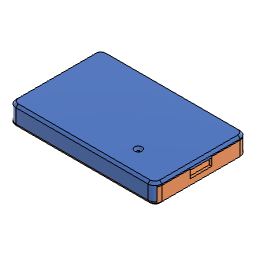
ESP32+Devkit+v4+Case (Autodesk Fusion 360 design; units mm, degrees)
Autodesk Fusion 360 part; units mm, degrees
sketch "Board" plane through (0, 0, 0) normal (0, 0, 1) x (1, 0, 0)
  line L0 (-24.2, 14.1) -> (24.2, 14.1)
  line L1 (24.2, 14.1) -> (24.2, -14.1)
  line L2 (24.2, -14.1) -> (-24.2, -14.1)
  line L3 (-24.2, -14.1) -> (-24.2, 14.1)
  line L4 (-24.2, 14.1) -> (24.2, -14.1) construction
  line L5 (24.2, 14.1) -> (-24.2, -14.1) construction
  line L6 (18.3, 3.8) -> (25, 3.8)
  line L7 (25, 3.8) -> (25, -3.8)
  line L8 (25, -3.8) -> (18.3, -3.8)
  line L9 (18.3, -3.8) -> (18.3, 3.8)
  line L10 (-24.2, 0) -> (24.2, 0) construction
  line L11 (-23.4, 7.9) -> (-5.9, 7.9)
  line L12 (-5.9, 7.9) -> (-5.9, -7.9)
  line L13 (-5.9, -7.9) -> (-23.4, -7.9)
  line L14 (-23.4, -7.9) -> (-23.4, 7.9)
  line L15 (-30.2, 9) -> (-23.4, 9)
  line L16 (-23.4, 9) -> (-23.4, -9)
  line L17 (-23.4, -9) -> (-30.2, -9)
  line L18 (-30.2, -9) -> (-30.2, 9)
  line L19 (-24, 14) -> (24, 14)
  line L20 (24, 14) -> (24, 11.6)
  line L21 (24, 11.6) -> (-24, 11.6)
  line L22 (-24, 11.6) -> (-24, 14)
  line L23 (-24, -11.6) -> (24, -11.6)
  line L24 (24, -11.6) -> (24, -14)
  line L25 (24, -14) -> (-24, -14)
  line L26 (-24, -14) -> (-24, -11.6)
  line L27 (10.2, -7.6) -> (12.2, -7.6)
  line L28 (12.2, -7.6) -> (12.2, -8.6)
  line L29 (12.2, -8.6) -> (10.2, -8.6)
  line L30 (10.2, -8.6) -> (10.2, -7.6)
  point P0 (25, 0)
  point P1 (-23.4, 0)
  dimension "d1" = 48.4
  dimension "d2" = 28.2
  dimension "d3" = 7.6
  dimension "d4" = 6.7
  dimension "d5" = 0.8
  dimension "d6" = 17.5
  dimension "d7" = 15.8
  dimension "d8" = 0.8
  dimension "d9" = 18
  dimension "d10" = 6.8
  dimension "d11" = 2.4
  dimension "d12" = 0.1
  dimension "d13" = 0.2
  dimension "d14" = 48
  dimension "d15" = 2.4
  dimension "d16" = 0.1
  dimension "d17" = 0.2
  dimension "d18" = 48
  dimension "d64" = 2
  dimension "d65" = 1
  dimension "d66" = 12
  dimension "d67" = 5.5
  constraint horizontal L0
  constraint perpendicular L0 L1
  constraint parallel L0 L2
  constraint parallel L1 L3
  constraint coincident L4 origin
  constraint coincident L5 origin
  constraint horizontal L6
  constraint vertical L7
  constraint horizontal L8
  constraint vertical L9
  constraint midpoint L3 L10.start
  constraint midpoint L1 L10.end
  constraint midpoint L7 P0
  constraint horizontal L10.end P0
  constraint horizontal L11
  constraint vertical L12
  constraint horizontal L13
  constraint vertical L14
  constraint midpoint L14 P1
  constraint horizontal L10.start P1
  constraint horizontal L15
  constraint vertical L16
  constraint horizontal L17
  constraint vertical L18
  constraint midpoint L14 L16
  constraint horizontal L19
  constraint vertical L20
  constraint horizontal L21
  constraint vertical L22
  constraint horizontal L23
  constraint vertical L24
  constraint horizontal L25
  constraint vertical L26
  constraint horizontal L27
  constraint vertical L28
  constraint horizontal L29
  constraint vertical L30
  measures "d1" distance of L0.start L0.end
  measures "d2" distance of L0.start L2.end
  measures "d3" distance of L6.end L7.end
  measures "d4" distance of L6.start L6.end
  measures "d5" distance of L1 L7
  measures "d6" distance of L11.start L11.end
  measures "d7" distance of L11.start L13.end
  measures "d8" distance of L3 L14
  measures "d9" distance of L15.start L17.end
  measures "d10" distance of L15.start L15.end
  measures "d11" distance of L19.end L20.end
  measures "d12" distance of L0 L19
  measures "d13" distance of L3 L22
  measures "d14" distance of L20.end L21.end
  measures "d15" distance of L23.end L24.end
  measures "d16" distance of L2 L25
  measures "d17" distance of L3 L26
  measures "d18" distance of L23.start L23.end
  measures "d64" distance of L27.start L27.end
  measures "d65" distance of L27.start L29.end
  measures "d66" distance of L1 L28.end
  measures "d67" distance of L2 L28.end
sketch "Case" plane through (0, 0, 0) normal (0, 0, 1) x (1, 0, 0)
  line L0 (-24.2, 14.1) -> (24.2, 14.1) construction
  line L1 (24.2, 14.1) -> (24.2, -14.1) construction
  line L2 (24.2, -14.1) -> (-24.2, -14.1) construction
  line L3 (-24.2, -14.1) -> (-24.2, 14.1) construction
  line L4 (24.4, -14.3) -> (-24.4, -14.3)
  line L5 (-24.4, -14.3) -> (-24.4, 14.3)
  line L6 (-24.4, 14.3) -> (24.4, 14.3)
  line L7 (24.4, 14.3) -> (24.4, -14.3)
  line L8 (25.3, -15.2) -> (-25.3, -15.2)
  line L9 (-25.3, -15.2) -> (-25.3, 15.2)
  line L10 (-25.3, 15.2) -> (25.3, 15.2)
  line L11 (25.3, 15.2) -> (25.3, -15.2)
  line L12 (26.4, -16.3) -> (-26.4, -16.3) construction
  line L13 (-26.4, -16.3) -> (-26.4, 16.3)
  line L14 (-26.4, 16.3) -> (26.4, 16.3) construction
  line L15 (26.4, 16.3) -> (26.4, -16.3) construction
  line L16 (25.3, 15.2) -> (25.3, 16.3)
  line L17 (25.3, -15.2) -> (25.3, -16.3)
  line L18 (25.3, 16.3) -> (-26.4, 16.3)
  line L19 (25.3, -16.3) -> (-26.4, -16.3)
  line L20 (24, 11.6) -> (-24, 11.6) construction
  line L21 (-24, -11.6) -> (24, -11.6) construction
  line L22 (-24.4, -11.4) -> (24.4, -11.4)
  line L23 (-24.4, 11.4) -> (24.4, 11.4)
  dimension "d26" = 0.2
  dimension "d27" = 0.2
  constraint coincident L14 L16.end
  constraint perpendicular L14 L16
  constraint coincident L12 L17.end
  constraint perpendicular L12 L17
  constraint coincident L5 L22.start
  constraint coincident L7 L22.end
  constraint perpendicular L7 L22
  constraint coincident L5 L23.start
  constraint coincident L7 L23.end
  constraint perpendicular L1 L23
  measures "d26" distance of L21 L22
  measures "d27" distance of L20 L23
extrude "Extrude1" add sketch "Case" against normal blind 1.2 contours L5 L7 L22 L23 | L8 L9 L10 L13 L16 L17 L18 L19 | L8 L9 L10 L11 makes body 1 in component "Base"
extrude "Extrude2" add sketch "Case" along normal blind 1.6 contours L8 L9 L10 L11 bodies 1 in component "Base"
sketch "Sketch3" plane through (0, 0, 1.6) normal (0, 0, 1) x (-1, 0, 0) in component "Base"
  line L0 (24.4, -14.3) -> (-24.4, -14.3)
  line L1 (-24.4, -14.3) -> (-24.4, 14.3)
  line L2 (-24.4, 14.3) -> (24.4, 14.3)
  line L3 (24.4, 14.3) -> (24.4, -14.3)
  line L4 (-25.3, -15.2) -> (25.3, -15.2)
  line L5 (25.3, -15.2) -> (25.3, 15.2)
  line L6 (25.3, 15.2) -> (-25.3, 15.2)
  line L7 (-25.3, 15.2) -> (-25.3, -15.2)
  line L8 (-18.3, -3.8) -> (-25, -3.8)
  line L9 (-25, 3.8) -> (-18.3, 3.8)
  line L10 (-25.3, -15.2) -> (-25.3, 15.2)
  line L11 (-24.4, -14.3) -> (-24.4, 14.3)
  line L12 (24.4, -14.3) -> (-24.4, -14.3)
  line L13 (25.3, -15.2) -> (-25.3, -15.2)
  line L14 (24.4, 14.3) -> (24.4, -14.3)
  line L15 (25.3, 15.2) -> (25.3, -15.2)
  line L16 (-24.4, 14.3) -> (24.4, 14.3)
  line L17 (-25.3, 15.2) -> (25.3, 15.2)
  line L18 (-24.4, -3.8) -> (-25.3, -3.8)
  line L19 (-24.4, 3.8) -> (-25.3, 3.8)
  line L20 (30.2, -9) -> (23.4, -9)
  line L21 (23.4, 9) -> (30.2, 9)
  constraint coincident L11 L18.start
  constraint coincident L8 L18.start
  constraint coincident L7 L18.end
  constraint perpendicular L7 L18
  constraint coincident L11 L19.start
  constraint coincident L9 L19.start
  constraint coincident L10 L19.end
  constraint perpendicular L10 L19
extrude "Extrude5" add sketch "Sketch3" along normal blind 3 contours L0 L1 L3 L4 L5 L7 L8 L10 L11 L12 L13 L14 L15 L18 L20 | L1 L2 L3 L5 L6 L7 L9 L10 L11 L14 L15 L16 L17 L19 L21 bodies 1 in component "Base"
fillet "Fillet1" radius 2.5 4 edges at (25.3, -16.3, -0.6) (25.3, 16.3, -0.6) (-26.4, -16.3, -0.6) (-26.4, 16.3, -0.6) on bodies 1 in component "Base"
chamfer "Chamfer1" distance 0.8 angle 45 8 edges at (25.3, 0, -1.2) (24.5678, -15.5678, -1.2) (-0.55, -16.3, -1.2) (-25.6678, -15.5678, -1.2) (-26.4, 0, -1.2) (-25.6678, 15.5678, -1.2) (-0.55, 16.3, -1.2) (24.5678, 15.5678, -1.2) on bodies 1 in component "Base"
sketch "Sketch4" plane through (25.3, 0, 0) normal (1, 0, 0) x (0, 1, 0)
  line L0 (-13.8, -0.4) -> (13.8, -0.4)
  line L1 (13.8, -0.4) -> (13.8, 4.6)
  line L2 (13.8, 4.6) -> (3.8, 4.6)
  line L3 (3.8, 4.6) -> (3.8, 1.6)
  line L4 (3.8, 1.6) -> (-3.8, 1.6)
  line L5 (-3.8, 1.6) -> (-3.8, 4.6)
  line L6 (-3.8, 4.6) -> (-13.8, 4.6)
  line L7 (-13.8, 4.6) -> (-13.8, -0.4)
  line L8 (-15.2, 4.6) -> (-15.2, 0)
  line L9 (-15.2, 2.3) -> (-15.6, 2.3) construction
  line L10 (-15.6, 2.3) -> (-15.2, 1.9)
  line L11 (-15.6, 2.3) -> (-15.2, 2.7)
  line L12 (-15.2, 2.7) -> (-15.2, 1.9)
  line L13 (15.2, 0) -> (15.2, 4.6)
  line L14 (15.2, 2.3) -> (15.6, 2.3) construction
  line L15 (15.6, 2.3) -> (15.2, 1.9)
  line L16 (15.6, 2.3) -> (15.2, 2.7)
  line L17 (15.2, 2.7) -> (15.2, 1.9)
  constraint midpoint L8 L9.start
  constraint perpendicular L8 L9
  constraint coincident L8 L10.end
  constraint coincident L8 L11.end
  constraint perpendicular L10 L11
  constraint midpoint L13 L14.start
  constraint perpendicular L13 L14
  constraint coincident L13 L15.end
  constraint coincident L13 L16.end
  constraint perpendicular L15 L16
extrude "Extrude6" add sketch "Sketch4" along normal blind -15 and the other way blind 35 contours L8 L10 L11 L12 | L13 L15 L16 L17 bodies 1 in component "Base"
extrude "Extrude1'" add sketch "Case" along normal blind 4.6 separate body contours L8 L9 L10 L13 L16 L17 L18 L19 makes body 2 in component "Lid"
sketch "Sketch1" plane through (0, 0, 4.6) normal (0, 0, 1) x (-1, 0, 0) in component "Lid"
  line L0 (-25.3, 15.2) -> (25.3, 15.2)
  line L1 (25.3, 15.2) -> (25.3, -15.2)
  line L2 (25.3, -15.2) -> (-25.3, -15.2)
  line L3 (-25.3, -15.2) -> (-25.3, -16.3)
  line L4 (-25.3, -16.3) -> (26.4, -16.3)
  line L5 (26.4, -16.3) -> (26.4, 16.3)
  line L6 (26.4, 16.3) -> (-25.3, 16.3)
  line L7 (-25.3, 16.3) -> (-25.3, 15.2)
  line L8 (26.4, -16.3) -> (-25.3, -16.3)
  line L9 (-25.3, -16.3) -> (-25.3, 16.3)
  line L10 (-25.3, 16.3) -> (26.4, 16.3)
  line L11 (26.4, 16.3) -> (26.4, -16.3)
  line L12 (25.3, 15.2) -> (25.3, -15.2)
  line L13 (-24.4, -14.3) -> (-24.4, 14.3)
  line L14 (-24.4, -3.8) -> (-25.3, -3.8)
  line L15 (-24.4, 3.8) -> (-25.3, 3.8)
  line L16 (30.2, -9) -> (23.4, -9)
  line L17 (23.4, 9) -> (30.2, 9)
  line L18 (-12.2, 8.6) -> (-10.2, 8.6)
  line L19 (-10.2, 7.6) -> (-12.2, 7.6)
  line L20 (-10.2, 8.6) -> (-10.2, 7.6)
  line L21 (-12.2, 7.6) -> (-12.2, 8.6)
  line L22 (-10.2, 7.6) -> (-12.2, 8.6) construction
  line L23 (-10.2, 8.6) -> (-12.2, 7.6) construction
  circle A0 centre (-11.2, 8.1) radius 0.5
  line L24 (23.4, -7.9) -> (5.9, -7.9) construction
  line L25 (5.9, -7.9) -> (5.9, 7.9) construction
  line L26 (5.9, 7.9) -> (23.4, 7.9) construction
  line L27 (23.4, 7.9) -> (23.4, -7.9) construction
  line L28 (23.6, -8.1) -> (5.7, -8.1)
  line L29 (5.7, -8.1) -> (5.7, 8.1)
  line L30 (5.7, 8.1) -> (23.6, 8.1)
  line L31 (23.6, 8.1) -> (23.6, -8.1)
  point P0 (23.4, -7.9)
  point P1 (5.9, 7.9)
  constraint horizontal L8
  constraint vertical L9
  constraint horizontal L10
  constraint vertical L11
  constraint coincident L6.end L7.start
  constraint coincident L4.end L5.start
  constraint coincident L19.start L20.end
  constraint coincident L18.start L21.end
  constraint coincident L18.end L20.start
  constraint coincident L19.end L21.start
  constraint midpoint L23 A0.centre
  constraint tangent L18 A0
  constraint horizontal L24
  constraint vertical L25
  constraint horizontal L26
  constraint vertical L27
  constraint coincident P1 L25.end
  constraint coincident P0 L24.start
extrude "Extrude2'" cut sketch "Sketch1" along normal blind -4.6 and the other way blind 1.6 contours L1 L5 L11 L12 L16 L17 bodies 2 in component "Lid"
extrude "Extrude3" add sketch "Sketch1" along normal blind 1.2 contours L0 L1 L5 L6 L7 L9 L10 L11 L12 L17 | L0 L1 L2 L9 L12 L13 L14 L15 | L9 L13 L14 L15 | L1 L5 L11 L12 L16 L17 | L1 L2 L3 L4 L5 L8 L9 L11 L12 L16 | L18 L19 L21 A0 | L18 L19 L20 A0 | A0 | L28 L29 L30 L31 bodies 2 in component "Lid"
extrude "Extrude4" add sketch "Sketch1" against normal blind 0.4 contours L9 L13 L14 L15 bodies 2 in component "Lid"
fillet "Fillet1'" radius 2.5 4 edges at (25.3, -16.3, 2.9) (25.3, 16.3, 2.9) (-26.4, -16.3, 2.9) (-26.4, 16.3, 2.9) on bodies 2 in component "Lid"
chamfer "Chamfer1'" distance 0.8 angle 45 8 edges at (-0.55, 16.3, 5.8) (-25.6678, 15.5678, 5.8) (-26.4, 0, 5.8) (-25.6678, -15.5678, 5.8) (-0.55, -16.3, 5.8) (24.5678, -15.5678, 5.8) (25.3, 0, 5.8) (24.5678, 15.5678, 5.8) on bodies 2 in component "Lid"
extrude "Extrude5'" cut sketch "Sketch4" along normal blind -15 and the other way blind 35 contours L8 L10 L11 L12 | L13 L15 L16 L17 bodies 2 in component "Lid"
extrude "Extrude6'" cut sketch "Sketch1" along normal blind 1.2 contours A0 bodies 2 in component "Lid"
chamfer "Chamfer2" distance 0.8 angle 45 1 edges at (11.6662, -8.2808, 5.8) on bodies 2 in component "Lid"
extrude "Extrude7" cut sketch "Sketch1" along normal blind 0.4 contours L28 L29 L30 L31 bodies 2 in component "Lid"
component "Base" placed x (1, 0, 0) y (0, 1, 0) z (0, 0, 1) at (0, 0, 0)
component "Lid" placed x (1, 0, 0) y (0, 1, 0) z (0, 0, 1) at (0, 0, 0)
equation "d19 = -fit_tollerance"
equation "inner_wall_thickness = 0.9 mm"
equation "outer_wall_thickness = 1.1 mm"
equation "base_thickness = 1.2 mm"
equation "fit_tollerance = 0.2 mm"
equation "d24 = -fit_tollerance - inner_wall_thickness"
equation "d25 = -fit_tollerance - inner_wall_thickness - outer_wall_thickness"
equation "d26 = fit_tollerance"
equation "d27 = fit_tollerance"
equation "d28 = -base_thickness"
equation "board_thickness = 1.6 mm"
equation "componnet_thickness = 3 mm"
equation "d32 = board_thickness"
equation "d38 = componnet_thickness"
equation "d43 = board_thickness + componnet_thickness"
equation "d45 = -componnet_thickness - board_thickness"
equation "d47 = componnet_thickness - 1.4 mm"
equation "d49 = base_thickness"
equation "d68 = base_thickness"
equation "d71 = -fit_tollerance"
